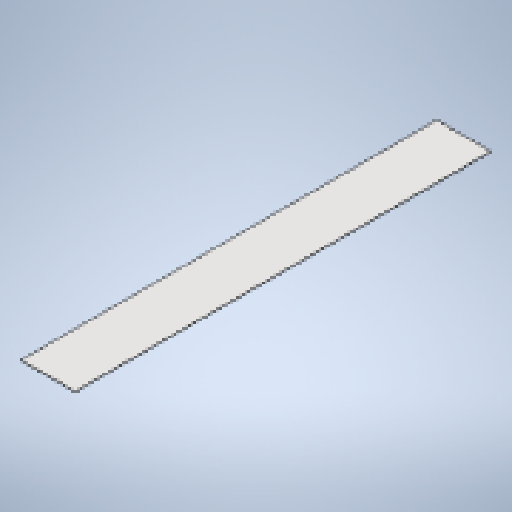
# Autodesk Inventor part: GnG L.5
Saved by Autodesk Inventor 2025 (Build 290162010, 162A)
## iProperties
Created: 2025-10-28
Part Number: GnG L.5
Material: Stainless Steel
Document SubType Name: Sheet Metal
Designer: admin
Mass: 280.619 g
Surface Area: 364.406 cm^2
Volume: 35.0774 cm^3
Density: 8 g/cm^3
Sheet Metal Rule: AISI304 3mm Die 32
Sheet Metal Width: 300,000 mm
Sheet Metal Length: 2300,000 mm
Sheet Metal Area: 690000,000 mm^2
Appearance: Default
Stock Number: L 5
Flat Pattern Width: 30 cm
Flat Pattern Length: 230 cm
Flat Pattern Area: 6900 cm^2
Author: admin
Autodesk Inventor part; units mm, degrees
ref_plane "YZ Plane" through (0, 0, 0) normal (1, 0, 0) x (0, 1, 0)
ref_plane "XZ Plane" through (0, 0, 0) normal (0, 1, 0) x (-1, 0, 0)
ref_plane "XY Plane" through (0, 0, 0) normal (0, 0, 1) x (1, 0, 0)
sketch "Sketch1" plane through (0, 0, 0) normal (0, 0, 1) x (1, 0, 0)
  line L0 (0, 0) -> (-300, 0)
  line L1 (-300, 0) -> (-300, -2300)
  line L2 (-300, -2300) -> (0, -2300)
  line L3 (0, -2300) -> (0, 0)
  line L4 (0, 0) -> (-40, 0)
  line L5 (-40, 0) -> (-40, -40)
  line L6 (-40, -40) -> (0, -40)
  line L7 (0, -40) -> (0, 0)
  line L8 (0, -2300) -> (-40, -2300)
  line L9 (-40, -2300) -> (-40, -2260)
  line L10 (-40, -2260) -> (0, -2260)
  line L11 (0, -2260) -> (0, -2300)
  line L12 (-300, 0) -> (-260, 0)
  line L13 (-260, 0) -> (-260, -40)
  line L14 (-260, -40) -> (-300, -40)
  line L15 (-300, -40) -> (-300, 0)
  line L16 (-300, -2300) -> (-260, -2300)
  line L17 (-260, -2300) -> (-260, -2260)
  line L18 (-260, -2260) -> (-300, -2260)
  line L19 (-300, -2260) -> (-300, -2300)
  line L20 (-220, -2300) -> (-130, -2300)
  line L21 (-130, -2300) -> (-130, -2260)
  line L22 (-130, -2260) -> (-220, -2260)
  line L23 (-220, -2260) -> (-220, -2300)
  line L24 (-220, 0) -> (-130, 0)
  line L25 (-130, 0) -> (-130, -40)
  line L26 (-130, -40) -> (-220, -40)
  line L27 (-220, -40) -> (-220, 0)
  point P0 (0, -40)
  point P1 (-40, 0)
  point P2 (-40, -2300)
  point P3 (0, -2260)
  point P4 (-130, 0)
  point P5 (-260, 0)
  point P6 (-300, -40)
  point P7 (-300, -2260)
  dimension "d22" = 300
  dimension "d23" = 2300
  dimension "d24" = 40
  dimension "d25" = 40
  dimension "d28" = 90
  dimension "d29" = 90
  measures "d22" distance of L2.end L1.end
  measures "d23" distance of L1.end L0.end
  measures "d24" distance of L6.end L5.end
  measures "d25" distance of L5.end L4.end
  measures "d28" distance of L25.end L26.end
  measures "d29" distance between parallel lines of L5 L25
extrude "Plate1" add sketch "Sketch1" along normal blind 3
sketch "Sketch5" plane through (0, 0, 3) normal (0, 0, 1) x (1, 0, 0)
  line L0 (0, -5) -> (0, 0) construction
  line L1 (-135, 0) -> (-231.2197, 0) construction
  line L2 (-231.2197, 0) -> (-236.2197, 0)
  line L3 (-236.2197, 0) -> (-236.2197, -2)
  line L4 (-236.2197, -2) -> (-231.2197, -2)
  line L5 (-231.2197, -2) -> (-231.2197, 0)
  circle A0 centre (-259.2728, 0) radius 2.5
  line L6 (-300, -2300) -> (0, -2300) projected
  line L7 (-300, 0) -> (-300, -2300) projected
  line L8 (0, 0) -> (-300, 0) projected
  line L9 (0, -2300) -> (0, 0) projected
  line L10 (0, 0) -> (-300, 0) projected
  line L11 (-221.2197, 0) -> (-226.2197, 0)
  line L12 (-226.2197, 0) -> (-226.2197, -2)
  line L13 (-226.2197, -2) -> (-221.2197, -2)
  line L14 (-221.2197, -2) -> (-221.2197, 0)
  line L15 (-211.2197, 0) -> (-216.2197, 0)
  line L16 (-216.2197, 0) -> (-216.2197, -2)
  line L17 (-216.2197, -2) -> (-211.2197, -2)
  line L18 (-211.2197, -2) -> (-211.2197, 0)
  line L19 (-201.2197, 0) -> (-206.2197, 0)
  line L20 (-206.2197, 0) -> (-206.2197, -2)
  line L21 (-206.2197, -2) -> (-201.2197, -2)
  line L22 (-201.2197, -2) -> (-201.2197, 0)
  line L23 (-191.2197, 0) -> (-196.2197, 0)
  line L24 (-196.2197, 0) -> (-196.2197, -2)
  line L25 (-196.2197, -2) -> (-191.2197, -2)
  line L26 (-191.2197, -2) -> (-191.2197, 0)
  dimension "d38" = 2
  dimension "d39" = 5
  dimension "d42" = 5
  dimension "d45" = 10
  constraints: 44 end point, 3 horizontal, 3 point on line, 2 parallel, 1 centre point, 1 coincident, 1 collinear, 1 perpendicular, 32 other
  measures "d38" distance of L3.end L2.end
  measures "d39" diameter of A0
  measures "d42" distance of L3.end L4.end
  measures "d45" distance of L1.end L11.start
extrude "Cut1" cut sketch "Sketch5" against normal blind 3 contours L5 L4 L3 L2 | L8 L14 L13 L12 | L8 A0 | A0 L8 | L8 L18 L17 L16 | L8 L22 L21 L20 | L8 L26 L25 L24
equation "\"d39\" = d32"
equation "\"d40\" = Thickness"
equation "\"d2\" = Thickness"
equation "\"BendReliefWidth\" = Thickness"
equation "\"BendReliefDepth\" = 0.5 * Thickness"
equation "\"CornerReliefSize\" = 4 * Thickness"
equation "\"MinimumRemnant\" = 2 * Thickness"
equation "\"TransitionRadius\" = BendRadius"
equation "\"JacobiRadiusSize\" = BendRadius"
equation "\"GapSize\" = Thickness"
equation "\"d32\" = 5"
equation "\"Thickness\" = 3"
equation "\"BendRadius\" = 5"
body "Solid1"
